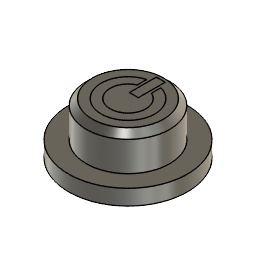
Mini PC Button V1 (Autodesk Fusion 360 design; units mm, degrees)
Autodesk Fusion 360 part; units mm, degrees
sketch "Sketch1" plane through (0, 0, 0) normal (0, 0, 1) x (1, 0, 0)
  circle A0 centre (0, 0) radius 5
  dimension "d1" = 10
  constraint coincident A0.centre origin
  measures "d1" diameter of A0
extrude "Extrude1" add sketch "Sketch1" along normal blind 1.3 makes body 1
sketch "Sketch2" plane through (0, 0, 1.3) normal (0, 0, 1) x (-1, 0, 0)
  circle A0 centre (0, 0) radius 5
  circle A1 centre (0, 0) radius 3.5
  dimension "d4" = 7
  constraint coincident A0.centre A1.centre
  measures "d4" diameter of A1
extrude "Extrude2" add sketch "Sketch2" along normal blind 3 contours A1 bodies 1
chamfer "Chamfer1" distance 0.5 angle 45 1 edges at (3.2631, 1.2657, 4.3) on bodies 1
sketch "Sketch3" plane through (0, 0, 4.3) normal (0, 0, 1) x (-1, 0, 0)
  circle A0 centre (0, 0) radius 3
  line L0 (-0.6, -1.3748) -> (-0.6, -2.1685)
  line L1 (0.6, -1.3748) -> (0.6, -2.1685)
  arc A1 (0.6, -1.3748) -> (-0.6, -1.3748) centre (0, 0) ccw
  arc A2 (0.6, -2.1685) -> (-0.6, -2.1685) centre (0, 0) ccw
  line L2 (0.375, -0.5) -> (-0.375, -0.5)
  line L3 (-0.375, -0.5) -> (-0.375, -2.75)
  line L4 (-0.375, -2.75) -> (0.375, -2.75)
  line L5 (0.375, -2.75) -> (0.375, -0.5)
  line L6 (0, 0) -> (0, -1) construction
  point P0 (0.6, -1)
  point P1 (-0.6, -1)
  dimension "d8" = 4.5
  dimension "d9" = 3
  dimension "d10" = 0.75
  dimension "d11" = 2.25
  constraint coincident A0.centre A1.centre
  constraint concentric A1 A2
  constraint vertical L0
  constraint parallel L0 L1
  constraint horizontal L2
  constraint vertical L3
  constraint horizontal L4
  constraint vertical L5
  constraint perpendicular L4 L6
  constraint midpoint L2 L6
  constraint vertical P1 L0.start
  constraint vertical P0 L1.start
  measures "d8" diameter of A2
  measures "d9" diameter of A1
  measures "d10" distance of L2.start L2.end
  measures "d11" distance of L2.start L4.end
extrude "Extrude3" add sketch "Sketch3" against normal blind 0.5 separate body contours L0 L1 A1 A2 | L2 L3 L4 L5 makes body 2 at (0.7039, 1.8668, 4.3) makes body 3 at (0.125, 1.25, 4.3)
combine "Combine1" operation cut target body 1 tool bodies 2 3 keep tools
